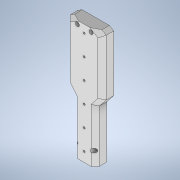
# Autodesk Inventor part: Deckel
Saved by Autodesk Inventor 2021 (Build 250183000, 183)
## iProperties
Created: 2024-05-18
Part Number: Deckel
Material: Generic
Document SubType Name: Modeling
Designer: Lukas
Density: 1 g/cm^3
Appearance: Default
Author: Lukas
Autodesk Inventor part; units mm, degrees
ref_plane "YZ Plane" through (0, 0, 0) normal (1, 0, 0) x (0, 1, 0)
ref_plane "XZ Plane" through (0, 0, 0) normal (0, 1, 0) x (-1, 0, 0)
ref_plane "XY Plane" through (0, 0, 0) normal (0, 0, 1) x (1, 0, 0)
sketch "Sketch1" plane through (0, 0, 0) normal (0, 0, 1) x (1, 0, 0)
  line L0 (-16, -130.2954) -> (-16, -53.8114)
  line L1 (-16, -53.8114) -> (-26.2, -41.0614)
  line L2 (-26.2, -41.0614) -> (-26.2, 41.0614)
  line L3 (16, -130.2954) -> (16, -53.8114)
  line L4 (16, -53.8114) -> (26.2, -41.0614)
  line L5 (26.2, -41.0614) -> (26.2, 41.0614)
  line L6 (-19.859, 44.9046) -> (19.859, 44.9046)
  line L7 (-26.2, 41.0614) -> (-19.859, 44.9046)
  line L8 (19.859, 44.9046) -> (26.2, 41.0614)
  line L9 (-16, -130.2954) -> (16, -130.2954)
  point P0 (0, 0)
  point P1 (0, 44.9046)
  point P2 (-26.2, 0)
  dimension "d0" = 76.484
  dimension "d1" = 32
  dimension "d3" = 10.2
  dimension "d4" = 12.75
  dimension "d8" = 85.966
  dimension "d9" = 39.718
  dimension "d10" = 148.78
  constraints: 20 end point, 3 equal length, 3 horizontal alignment, 2 horizontal, 2 midpoint, 2 parallel, 2 vertical, 1 vertical alignment
  measures "d0" distance of L0.start L0.end
  measures "d1" distance between parallel lines of L3 L0
  measures "d3" horizontal distance of L0.end L1.end
  measures "d4" vertical distance of L0.end L1.end
  measures "d8" distance from line of L6 L1.end
  measures "d9" distance of L6.start L6.end
  measures "d10" angle of L6 L7
extrude "Extrusion1" add sketch "Sketch1" along normal blind 17
sketch "Sketch3" plane through (0, 0, 0) normal (0, 0, -1) x (-1, 0, 0)
  line L0 (16, -53.8114) -> (16, -130.2954) projected
  line L1 (26.2, -41.0614) -> (16, -53.8114) projected
  line L2 (26.2, 41.0614) -> (26.2, -41.0614) projected
  line L3 (19.859, 44.9046) -> (26.2, 41.0614) projected
  line L4 (-19.859, 44.9046) -> (19.859, 44.9046) projected
  line L5 (-26.2, 41.0614) -> (-19.859, 44.9046) projected
  line L6 (-26.2, -41.0614) -> (-26.2, 41.0614) projected
  line L7 (-16, -53.8114) -> (-26.2, -41.0614) projected
  line L8 (-16, -130.2954) -> (-16, -53.8114) projected
  line L9 (23.2, -40.009) -> (13, -52.759)
  line L10 (13, -52.759) -> (13, -127.2954)
  line L11 (-13, -127.2954) -> (-13, -52.759)
  line L12 (-13, -52.759) -> (-23.2, -40.009)
  line L13 (-23.2, -40.009) -> (-23.2, 39.3716)
  line L14 (-23.2, 39.3716) -> (-19.0208, 41.9046)
  line L15 (-19.0208, 41.9046) -> (19.0208, 41.9046)
  line L16 (19.0208, 41.9046) -> (23.2, 39.3716)
  line L17 (23.2, 39.3716) -> (23.2, -40.009)
  line L18 (13, -127.2954) -> (-13, -127.2954)
  line L19 (16, -130.2954) -> (-16, -130.2954) projected
  point P0 (0, 0)
  dimension "d22" = 3
  dimension "d108" = 3
  dimension "d109" = 3
  constraints: 20 end point, 7 other
  measures "d22" distance between parallel lines of L2 L17
  measures "d108" distance between parallel lines of L1 L9
  measures "d109" distance between parallel lines of L19 L18
extrude "Extrusion3" cut sketch "Sketch3" against normal blind 15 contours L9 L10 L18 L11 L12 L13 L14 L15 L16 L17
sketch "Sketch4" plane through (0, 0, 0) normal (0, 0, -1) x (-1, 0, 0)
  circle A0 centre (-12, -110.2954) radius 1.6
  circle A1 centre (12, -110.2954) radius 1.6
  circle A2 centre (12, -110.2954) radius 4
  circle A3 centre (-12, -110.2954) radius 4
  line L0 (-13, -127.2954) -> (-13, -52.759) projected
  line L1 (13, -52.759) -> (13, -127.2954) projected
  circle A4 centre (10, 39.9046) radius 1.6
  circle A5 centre (-10, 39.9046) radius 1.6
  line L2 (-19.859, 44.9046) -> (19.859, 44.9046) projected
  circle A6 centre (-10, 39.9046) radius 4
  circle A7 centre (10, 39.9046) radius 4
  line L3 (-19.0208, 41.9046) -> (19.0208, 41.9046) projected
  line L4 (16, -130.2954) -> (-16, -130.2954) projected
  point P0 (0, 0)
  point P1 (0, -114.2954)
  point P2 (12, -114.2954)
  point P3 (12.039, -111.8949)
  point P4 (12.091, -108.698)
  point P5 (12.13, -106.2975)
  point P6 (-12.13, -106.2975)
  point P7 (-12.091, -108.698)
  point P8 (-12.039, -111.8949)
  point P9 (-12, -114.2954)
  point P10 (-6.5359, 41.9046)
  point P11 (-8.751, 40.9046)
  point P12 (-11.249, 40.9046)
  point P13 (-13.4641, 41.9046)
  point P14 (13.4641, 41.9046)
  point P15 (11.249, 40.9046)
  point P16 (8.751, 40.9046)
  point P17 (6.5359, 41.9046)
  point P18 (-13, -114.2954)
  point P19 (13, -114.2954)
  point P20 (13, -111.5444)
  point P21 (13, -109.0464)
  point P22 (13, -114.1683)
  point P23 (13, -106.4224)
  point P24 (-13, -109.0464)
  point P25 (-13, -111.5444)
  point P26 (-13, -106.4224)
  point P27 (-13, -114.1683)
  dimension "d28" = 3.2
  dimension "d30" = 12
  dimension "d31" = 12
  dimension "d32" = 8
  dimension "d40" = 5
  dimension "d41" = 3.2
  dimension "d42" = 10
  dimension "d43" = 20
  dimension "d44" = 8
  dimension "d107" = 20
  constraints: 8 centre point, 4 coincident, 4 equal radius, 2 horizontal alignment
  measures "d28" diameter of A0
  measures "d30" horizontal distance of A1.centre point (0, -114.295)
  measures "d31" horizontal distance of point (0, -114.295) A0.centre
  measures "d32" diameter of A3
  measures "d40" distance from line of L2 A5.centre
  measures "d41" diameter of A5
  measures "d42" horizontal distance of point (0, 0) A5.centre
  measures "d43" distance of A4.centre A5.centre
  measures "d44" diameter of A6
  measures "d107" distance from line of L4 A2.centre
extrude "Extrusion4" cut sketch "Sketch4" against normal through all contours A0 L0 | L0 A0 | A1 L1 | L1 A1 | A4 | A5
extrude "Extrusion5" add sketch "Sketch4" against normal up to surface (15 mm away) contours A0 L0 A3 | A1 L1 A2 | A6 L3 | A7 L3 picked at (-8.8345, -110.5967) picked at (12.4395, -107.146) picked at (-10.0643, 41.7674) picked at (9.9357, 41.7674)
chamfer "Chamfer2" distance 4 angle 45 17 edges at (-18.1, -46.384, 15) (-23.2, -0.3187, 15) (-13, -79.5907, 15) (13, -79.5907, 15) (18.1, -46.384, 15) (23.2, -0.3187, 15) (21.1104, 40.6381, 15) (16.2425, 41.9046, 15) (10, 35.9046, 15) (0, 41.9046, 15) (-10, 35.9046, 15) (-16.2425, 41.9046, 15) (-21.1104, 40.6381, 15) (8, -110.2954, 15) (-8, -110.2954, 15) (13, -120.7319, 15) (-13, -120.7319, 15)
chamfer "Chamfer1" distance 6 angle 45 8 edges at (-16, -92.0534, 17) (16, -92.0534, 17) (21.1, -47.4364, 17) (-21.1, -47.4364, 17) (-26.2, 0, 17) (26.2, 0, 17) (23.0295, 42.983, 17) (-23.0295, 42.983, 17)
sketch "Sketch5" plane through (0, 0, 17) normal (0, 0, 1) x (1, 0, 0)
  circle A0 centre (-12, -110.2954) radius 1.6 projected
  circle A1 centre (-12, -110.2954) radius 1.6 projected
  circle A2 centre (12, -110.2954) radius 1.6 projected
  circle A3 centre (12, -110.2954) radius 1.6 projected
  circle A4 centre (-12, -110.2954) radius 3
  circle A5 centre (12, -110.2954) radius 3
  circle A6 centre (-10, 39.9046) radius 1.6 projected
  circle A7 centre (10, 39.9046) radius 1.6 projected
  circle A8 centre (-10, 39.9046) radius 3
  circle A9 centre (10, 39.9046) radius 3
  point P0 (0, 0)
  dimension "d37" = 6
  constraints: 4 centre point, 3 equal radius, 2 coincident
  measures "d37" diameter of A4
extrude "Extrusion6" cut sketch "Sketch5" along normal blind 13 and the other way blind 6.5 contours A0 | A2 | A4 | A5 | A6 | A7 | A8 | A9
fillet "Fillet1" radius 2 6 edges at (13, -106.4224, 5.5) (-13, -106.4224, 5.5) (6.5359, 41.9046, 5.5) (13.4641, 41.9046, 5.5) (-13.4641, 41.9046, 5.5) (-6.5359, 41.9046, 5.5)
sketch "Sketch13" plane through (0, 0, 17) normal (0, 0, 1) x (1, 0, 0)
  circle A0 centre (0, -116.2954) radius 1.4
  circle A1 centre (0, -56.2954) radius 1.4
  circle A2 centre (0, -86.2954) radius 1.4
  circle A3 centre (0, -26.2954) radius 1.4
  line L0 (8.2833, 44.9046) -> (-8.2833, 44.9046) projected
  circle A4 centre (0, 3.7046) radius 1.4
  circle A5 centre (0, 33.7046) radius 1.4
  line L1 (-10, -130.2954) -> (10, -130.2954) projected
  point P0 (0, 0)
  dimension "d96" = 2.8
  dimension "d99" = 30
  dimension "d100" = 30
  dimension "d101" = 30
  dimension "d102" = 30
  dimension "d103" = 30
  dimension "d110" = 14
  constraints: 6 centre point, 6 vertical alignment, 5 equal radius
  measures "d96" diameter of A0
  measures "d99" distance of A0.centre A2.centre
  measures "d100" distance of A1.centre A2.centre
  measures "d101" distance of A3.centre A1.centre
  measures "d102" distance of A3.centre A4.centre
  measures "d103" distance of A5.centre A4.centre
  measures "d110" distance from line of L1 A0.centre
extrude "Extrusion13" cut sketch "Sketch13" against normal through all
sketch "Sketch14" plane through (-16, -130.2954, 0) normal (0, -1, 0) x (1, 0, 0)
  circle A0 centre (8, 8) radius 1.4
  circle A1 centre (24, 8) radius 1.4
  line L0 (0, 0) -> (32, 0) projected
  point P0 (16, 0)
  dimension "d111" = 8
  dimension "d112" = 8
  dimension "d113" = 8
  dimension "d114" = 2.8
  constraints: 2 centre point, 1 equal radius, 1 horizontal alignment
  measures "d111" distance from line of L0 A1.centre
  measures "d112" horizontal distance of point (16, 0) A0.centre
  measures "d113" horizontal distance of A1.centre point (16, 0)
  measures "d114" diameter of A0
extrude "Extrusion14" cut sketch "Sketch14" against normal blind 5
equation "\"d31\" = d30"
equation "\"d43\" = 2 * d42"
body "Solid1"
